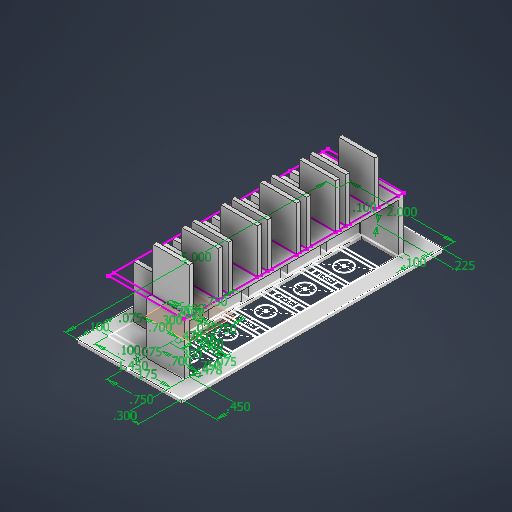
# Autodesk Inventor part: SolenoidHolders
Saved by Autodesk Inventor 2026.2 (Build 302298010, 298A)
## iProperties
Created: 2026-03-29
Part Number: SolenoidHolders
Material: Generic
Document SubType Name: Modeling
Designer: david
Density: 1 g/cm^3
Appearance: Default
Author: david
Autodesk Inventor part; units mm, degrees
ref_plane "YZ Plane" through (0, 0, 0) normal (1, 0, 0) x (0, 1, 0)
ref_plane "XZ Plane" through (0, 0, 0) normal (0, 1, 0) x (-1, 0, 0)
ref_plane "XY Plane" through (0, 0, 0) normal (0, 0, 1) x (1, 0, 0)
sketch "Sketch2" plane through (0, 0, 0) normal (0, 1, 0) x (-1, 0, 0)
  line L0 (0, 0) -> (17.78, 0)
  line L1 (17.78, 0) -> (17.78, -1.905)
  line L2 (17.78, -1.905) -> (0, -1.905)
  line L3 (0, -1.905) -> (0, 0)
  line L4 (17.78, -1.905) -> (0, -1.905)
  line L5 (0, -1.905) -> (0, -14.0462)
  line L6 (0, -14.0462) -> (17.78, -14.0462)
  line L7 (17.78, -14.0462) -> (17.78, -1.905)
  line L8 (17.78, -14.0462) -> (0, -14.0462)
  line L9 (0, -14.0462) -> (0, -15.9512)
  line L10 (0, -15.9512) -> (17.78, -15.9512)
  line L11 (17.78, -15.9512) -> (17.78, -14.0462)
  circle A0 centre (8.89, -7.9756) radius 3.81
  line L12 (17.78, -1.905) -> (0, -14.0462) construction
  line L13 (0, -19.05) -> (17.78, -19.05)
  line L14 (17.78, -19.05) -> (17.78, -20.955)
  line L15 (17.78, -20.955) -> (0, -20.955)
  line L16 (0, -20.955) -> (0, -19.05)
  line L17 (17.78, -20.955) -> (0, -20.955)
  line L18 (0, -20.955) -> (0, -33.0962)
  line L19 (0, -33.0962) -> (17.78, -33.0962)
  line L20 (17.78, -33.0962) -> (17.78, -20.955)
  line L21 (17.78, -33.0962) -> (0, -33.0962)
  line L22 (0, -33.0962) -> (0, -35.0012)
  line L23 (0, -35.0012) -> (17.78, -35.0012)
  line L24 (17.78, -35.0012) -> (17.78, -33.0962)
  circle A1 centre (8.89, -27.0256) radius 3.81
  line L25 (17.78, -20.955) -> (0, -33.0962) construction
  line L26 (0, -38.1) -> (17.78, -38.1)
  line L27 (17.78, -38.1) -> (17.78, -40.005)
  line L28 (17.78, -40.005) -> (0, -40.005)
  line L29 (0, -40.005) -> (0, -38.1)
  line L30 (17.78, -40.005) -> (0, -40.005)
  line L31 (0, -40.005) -> (0, -52.1462)
  line L32 (0, -52.1462) -> (17.78, -52.1462)
  line L33 (17.78, -52.1462) -> (17.78, -40.005)
  line L34 (17.78, -52.1462) -> (0, -52.1462)
  line L35 (0, -52.1462) -> (0, -54.0512)
  line L36 (0, -54.0512) -> (17.78, -54.0512)
  line L37 (17.78, -54.0512) -> (17.78, -52.1462)
  circle A2 centre (8.89, -46.0756) radius 3.81
  line L38 (17.78, -40.005) -> (0, -52.1462) construction
  line L39 (0, -57.15) -> (17.78, -57.15)
  line L40 (17.78, -57.15) -> (17.78, -59.055)
  line L41 (17.78, -59.055) -> (0, -59.055)
  line L42 (0, -59.055) -> (0, -57.15)
  line L43 (17.78, -59.055) -> (0, -59.055)
  line L44 (0, -59.055) -> (0, -71.1962)
  line L45 (0, -71.1962) -> (17.78, -71.1962)
  line L46 (17.78, -71.1962) -> (17.78, -59.055)
  line L47 (17.78, -71.1962) -> (0, -71.1962)
  line L48 (0, -71.1962) -> (0, -73.1012)
  line L49 (0, -73.1012) -> (17.78, -73.1012)
  line L50 (17.78, -73.1012) -> (17.78, -71.1962)
  circle A3 centre (8.89, -65.1256) radius 3.81
  line L51 (17.78, -59.055) -> (0, -71.1962) construction
  line L52 (0, -76.2) -> (17.78, -76.2)
  line L53 (17.78, -76.2) -> (17.78, -78.105)
  line L54 (17.78, -78.105) -> (0, -78.105)
  line L55 (0, -78.105) -> (0, -76.2)
  line L56 (17.78, -78.105) -> (0, -78.105)
  line L57 (0, -78.105) -> (0, -90.2462)
  line L58 (0, -90.2462) -> (17.78, -90.2462)
  line L59 (17.78, -90.2462) -> (17.78, -78.105)
  line L60 (17.78, -90.2462) -> (0, -90.2462)
  line L61 (0, -90.2462) -> (0, -92.1512)
  line L62 (0, -92.1512) -> (17.78, -92.1512)
  line L63 (17.78, -92.1512) -> (17.78, -90.2462)
  circle A4 centre (8.89, -84.1756) radius 3.81
  line L64 (17.78, -78.105) -> (0, -90.2462) construction
  line L65 (-7.62, 11.43) -> (43.18, 11.43)
  line L66 (43.18, 11.43) -> (43.18, -115.57)
  line L67 (43.18, -115.57) -> (-7.62, -115.57)
  line L68 (-7.62, -115.57) -> (-7.62, 11.43)
  line L69 (19.05, -9.525) -> (36.83, -9.525)
  line L70 (36.83, -9.525) -> (36.83, -11.43)
  line L71 (36.83, -11.43) -> (19.05, -11.43)
  line L72 (19.05, -11.43) -> (19.05, -9.525)
  line L73 (36.83, -11.43) -> (19.05, -11.43)
  line L74 (19.05, -11.43) -> (19.05, -23.5712)
  line L75 (19.05, -23.5712) -> (36.83, -23.5712)
  line L76 (36.83, -23.5712) -> (36.83, -11.43)
  line L77 (36.83, -23.5712) -> (19.05, -23.5712)
  line L78 (19.05, -23.5712) -> (19.05, -25.4762)
  line L79 (19.05, -25.4762) -> (36.83, -25.4762)
  line L80 (36.83, -25.4762) -> (36.83, -23.5712)
  circle A5 centre (27.94, -17.5006) radius 3.81
  line L81 (36.83, -11.43) -> (19.05, -23.5712) construction
  line L82 (19.05, -28.575) -> (36.83, -28.575)
  line L83 (36.83, -28.575) -> (36.83, -30.48)
  line L84 (36.83, -30.48) -> (19.05, -30.48)
  line L85 (19.05, -30.48) -> (19.05, -28.575)
  line L86 (36.83, -30.48) -> (19.05, -30.48)
  line L87 (19.05, -30.48) -> (19.05, -42.6212)
  line L88 (19.05, -42.6212) -> (36.83, -42.6212)
  line L89 (36.83, -42.6212) -> (36.83, -30.48)
  line L90 (36.83, -42.6212) -> (19.05, -42.6212)
  line L91 (19.05, -42.6212) -> (19.05, -44.5262)
  line L92 (19.05, -44.5262) -> (36.83, -44.5262)
  line L93 (36.83, -44.5262) -> (36.83, -42.6212)
  circle A6 centre (27.94, -36.5506) radius 3.81
  line L94 (36.83, -30.48) -> (19.05, -42.6212) construction
  line L95 (19.05, -47.625) -> (36.83, -47.625)
  line L96 (36.83, -47.625) -> (36.83, -49.53)
  line L97 (36.83, -49.53) -> (19.05, -49.53)
  line L98 (19.05, -49.53) -> (19.05, -47.625)
  line L99 (36.83, -49.53) -> (19.05, -49.53)
  line L100 (19.05, -49.53) -> (19.05, -61.6712)
  line L101 (19.05, -61.6712) -> (36.83, -61.6712)
  line L102 (36.83, -61.6712) -> (36.83, -49.53)
  line L103 (36.83, -61.6712) -> (19.05, -61.6712)
  line L104 (19.05, -61.6712) -> (19.05, -63.5762)
  line L105 (19.05, -63.5762) -> (36.83, -63.5762)
  line L106 (36.83, -63.5762) -> (36.83, -61.6712)
  circle A7 centre (27.94, -55.6006) radius 3.81
  line L107 (36.83, -49.53) -> (19.05, -61.6712) construction
  line L108 (19.05, -66.675) -> (36.83, -66.675)
  line L109 (36.83, -66.675) -> (36.83, -68.58)
  line L110 (36.83, -68.58) -> (19.05, -68.58)
  line L111 (19.05, -68.58) -> (19.05, -66.675)
  line L112 (36.83, -68.58) -> (19.05, -68.58)
  line L113 (19.05, -68.58) -> (19.05, -80.7212)
  line L114 (19.05, -80.7212) -> (36.83, -80.7212)
  line L115 (36.83, -80.7212) -> (36.83, -68.58)
  line L116 (36.83, -80.7212) -> (19.05, -80.7212)
  line L117 (19.05, -80.7212) -> (19.05, -82.6262)
  line L118 (19.05, -82.6262) -> (36.83, -82.6262)
  line L119 (36.83, -82.6262) -> (36.83, -80.7212)
  circle A8 centre (27.94, -74.6506) radius 3.81
  line L120 (36.83, -68.58) -> (19.05, -80.7212) construction
  line L121 (19.05, -85.725) -> (36.83, -85.725)
  line L122 (36.83, -85.725) -> (36.83, -87.63)
  line L123 (36.83, -87.63) -> (19.05, -87.63)
  line L124 (19.05, -87.63) -> (19.05, -85.725)
  line L125 (36.83, -87.63) -> (19.05, -87.63)
  line L126 (19.05, -87.63) -> (19.05, -99.7712)
  line L127 (19.05, -99.7712) -> (36.83, -99.7712)
  line L128 (36.83, -99.7712) -> (36.83, -87.63)
  line L129 (36.83, -99.7712) -> (19.05, -99.7712)
  line L130 (19.05, -99.7712) -> (19.05, -101.6762)
  line L131 (19.05, -101.6762) -> (36.83, -101.6762)
  line L132 (36.83, -101.6762) -> (36.83, -99.7712)
  circle A9 centre (27.94, -93.7006) radius 3.81
  line L133 (36.83, -87.63) -> (19.05, -99.7712)
  line L134 (8.89, -15.9512) -> (8.89, -19.05) construction
  line L135 (0, 0) -> (36.83, 0)
  line L136 (36.83, 0) -> (36.83, 2.54)
  line L137 (36.83, 2.54) -> (0, 2.54)
  line L138 (0, 2.54) -> (0, 0)
  line L139 (36.83, -101.6762) -> (0, -101.6762)
  line L140 (0, -101.6762) -> (0, -104.2162)
  line L141 (0, -104.2162) -> (36.83, -104.2162)
  line L142 (36.83, -104.2162) -> (36.83, -101.6762)
  circle A10 centre (18.415, 6.985) radius 1.27
  line L143 (19.05, -9.525) -> (17.78, -9.525) construction
  line L144 (19.05, -10.4775) -> (17.78, -10.4775) construction
  circle A11 centre (18.415, -109.855) radius 1.27
  line L145 (22.86, -25.4762) -> (22.86, -28.575)
  line L146 (22.86, -28.575) -> (33.02, -28.575)
  line L147 (33.02, -28.575) -> (33.02, -25.4762)
  line L148 (33.02, -25.4762) -> (22.86, -25.4762)
  line L149 (22.86, -25.4762) -> (33.02, -28.575) construction
  line L150 (22.86, -28.575) -> (33.02, -25.4762) construction
  line L151 (22.86, -47.625) -> (33.02, -47.625)
  line L152 (33.02, -44.5262) -> (22.86, -44.5262)
  line L153 (22.86, -44.5262) -> (22.86, -47.625)
  line L154 (33.02, -47.625) -> (33.02, -44.5262)
  line L155 (22.86, -44.5262) -> (33.02, -47.625) construction
  line L156 (22.86, -47.625) -> (33.02, -44.5262) construction
  line L157 (22.86, -66.675) -> (33.02, -66.675)
  line L158 (33.02, -63.5762) -> (22.86, -63.5762)
  line L159 (22.86, -63.5762) -> (22.86, -66.675)
  line L160 (33.02, -66.675) -> (33.02, -63.5762)
  line L161 (22.86, -63.5762) -> (33.02, -66.675) construction
  line L162 (22.86, -66.675) -> (33.02, -63.5762) construction
  line L163 (22.86, -85.725) -> (33.02, -85.725)
  line L164 (33.02, -82.6262) -> (22.86, -82.6262)
  line L165 (22.86, -82.6262) -> (22.86, -85.725)
  line L166 (33.02, -85.725) -> (33.02, -82.6262)
  line L167 (22.86, -82.6262) -> (33.02, -85.725) construction
  line L168 (22.86, -85.725) -> (33.02, -82.6262) construction
  line L169 (3.81, -15.9512) -> (3.81, -19.05)
  line L170 (3.81, -19.05) -> (13.97, -19.05)
  line L171 (13.97, -19.05) -> (13.97, -15.9512)
  line L172 (13.97, -15.9512) -> (3.81, -15.9512)
  line L173 (3.81, -15.9512) -> (13.97, -19.05) construction
  line L174 (3.81, -19.05) -> (13.97, -15.9512) construction
  line L175 (3.81, -38.1) -> (13.97, -38.1)
  line L176 (13.97, -35.0012) -> (3.81, -35.0012)
  line L177 (3.81, -35.0012) -> (13.97, -38.1) construction
  line L178 (3.81, -38.1) -> (13.97, -35.0012) construction
  line L179 (3.81, -35.0012) -> (3.81, -38.1)
  line L180 (13.97, -38.1) -> (13.97, -35.0012)
  line L181 (8.89, -35.0012) -> (8.89, -38.1) construction
  line L182 (3.81, -57.15) -> (13.97, -57.15)
  line L183 (13.97, -54.0512) -> (3.81, -54.0512)
  line L184 (3.81, -54.0512) -> (13.97, -57.15) construction
  line L185 (3.81, -57.15) -> (13.97, -54.0512) construction
  line L186 (3.81, -54.0512) -> (3.81, -57.15)
  line L187 (13.97, -57.15) -> (13.97, -54.0512)
  line L188 (8.89, -54.0512) -> (8.89, -57.15) construction
  line L189 (3.81, -76.2) -> (13.97, -76.2)
  line L190 (13.97, -73.1012) -> (3.81, -73.1012)
  line L191 (3.81, -73.1012) -> (13.97, -76.2) construction
  line L192 (3.81, -76.2) -> (13.97, -73.1012) construction
  line L193 (3.81, -73.1012) -> (3.81, -76.2)
  line L194 (13.97, -76.2) -> (13.97, -73.1012)
  line L195 (8.89, -73.1012) -> (8.89, -76.2) construction
  line L196 (0, 0) -> (17.78, 0)
  line L197 (17.78, 0) -> (17.78, -101.6762)
  line L198 (17.78, -101.6762) -> (0, -101.6762)
  line L199 (0, -101.6762) -> (0, 0)
  line L200 (36.83, 0) -> (0, 0)
  line L201 (0, 0) -> (0, -101.6762)
  line L202 (0, -101.6762) -> (36.83, -101.6762)
  line L203 (36.83, -101.6762) -> (36.83, 0)
  line L204 (18.415, 2.54) -> (18.415, 0)
  line L205 (18.415, -101.6762) -> (18.415, -104.2162)
  point P0 (8.89, -17.5006)
  point P1 (18.415, -10.4775)
  point P2 (17.78, 11.43)
  point P3 (31.0864, -91.5521)
  point P4 (24.7936, -95.8491)
  point P5 (27.94, -27.0256)
  point P6 (27.94, -27.0256)
  point P7 (27.94, -46.0756)
  point P8 (27.94, -46.0756)
  point P9 (27.94, -65.1256)
  point P10 (27.94, -65.1256)
  point P11 (27.94, -84.1756)
  point P12 (27.94, -84.1756)
  point P13 (8.89, -36.5506)
  point P14 (8.89, -55.6006)
  point P15 (8.89, -74.6506)
  dimension "d68" = 17.78
  dimension "d69" = 1.905
  dimension "d70" = 17.78
  dimension "d71" = 12.1412
  dimension "d72" = 17.78
  dimension "d73" = 1.905
  dimension "d74" = 7.62
  dimension "d77" = 19.05
  dimension "d82" = 50.8
  dimension "d83" = 127
  dimension "d84" = 11.43
  dimension "d85" = 7.62
  dimension "d90" = 17.78
  dimension "d91" = 1.905
  dimension "d92" = 17.78
  dimension "d93" = 12.1412
  dimension "d94" = 17.78
  dimension "d95" = 1.905
  dimension "d96" = 7.62
  dimension "d97" = 19.05
  dimension "d99" = 19.05
  dimension "d100" = 36.83
  dimension "d101" = 2.54
  dimension "d102" = 2.54
  dimension "d103" = 2.54
  dimension "d104" = 4.445
  dimension "d105" = 2.54
  dimension "d106" = 5.715
  dimension "d113" = 10.16
  dimension "d114" = 3.0988
  dimension "d117" = 19.05
  dimension "d122" = 10.16
  dimension "d125" = 19.05
  constraints: 412 end point, 29 midpoint, 26 parallel, 17 perpendicular, 12 centre point, 11 horizontal, 10 coincident, 6 collinear, 4 vertical, 3 point on line, 3 vertical alignment, 1 horizontal alignment, 284 other
  measures "d68" distance of L1.end L2.end
  measures "d69" distance of L0.end L1.end
  measures "d70" distance of L6.end L5.end
  measures "d71" distance of L5.end L4.end
  measures "d72" distance of L10.end L9.end
  measures "d73" distance of L9.end L8.end
  measures "d74" diameter of A0
  measures "d77" distance of L0.start L13.start
  measures "d82" distance of L66.end L67.end
  measures "d83" distance of L65.end L66.end
  measures "d84" distance between parallel lines of L0 L65
  measures "d85" distance from line of L0.start L68
  measures "d90" distance of L71.start L71.end
  measures "d91" distance of L69.end L71.start
  measures "d92" distance of L75.end L74.end
  measures "d93" distance of L74.end L73.end
  measures "d94" distance of L79.end L78.end
  measures "d95" distance of L78.end L77.end
  measures "d96" diameter of A5
  measures "d97" distance of L69.start L82.start
  measures "d99" distance between parallel lines of L18 L74
  measures "d100" distance of L137.end L136.end
  measures "d101" distance of L136.end L135.end
  measures "d102" distance of L140.end L139.end
  measures "d103" diameter of A10
  measures "d104" vertical distance of point (17.78, 11.43) A10.centre
  measures "d105" diameter of A11
  measures "d106" distance from line of L67 A11.centre
  measures "d113" distance of L146.end L145.end
  measures "d114" distance between parallel lines of L146 L148
  measures "d117" distance of L145.end L151.start
  measures "d122" distance of L170.end L169.end
  measures "d125" distance of L170.end L175.end
extrude "Extrusion1" add sketch "Sketch2" against normal blind 1.905 contours L138 L137 L204 L135 L0 | L135 L203 L69 L72 L74 L78 L79 L145 L82 L85 L87 L91 L92 L153 L95 L98 L100 L104 L105 L159 L108 L111 L113 L117 L118 L165 L121 L124 L126 L130 L139 L197 L63 L59 L53 L50 L46 L40 L37 L33 L27 L24 L20 L14 L11 L7 L1 | L204 L137 L136 L135 | L70 L71 L72 L69 | L76 L75 L74 L71 | L80 L79 L78 L75 | L203 L82 L147 L79 | L147 L82 L145 L79 | L83 L84 L85 L82 | L89 L88 L87 L84 | L93 L92 L91 L88 | L203 L95 L154 L92 | L154 L95 L153 L92 | L96 L97 L98 L95 | L102 L101 L100 L97 | L106 L105 L104 L101 | L203 L108 L160 L105 | L160 L108 L159 L105 | L109 L110 L111 L108 | L115 L114 L113 L110 | L119 L118 L117 L114 | L203 L121 L166 L118 | L166 L121 L165 L118 | L122 L123 L124 L121 | L139 L205 L141 L140 | L133 A9 L126 L123 | L128 L127 L133 A9 | L139 L131 L142 L141 L205 | L132 L131 L130 L127 | L133 A9 | A9 L133 | L65 L66 L67 L68 | A5 | A6 | A7 | A8
extrude "Extrusion2" add sketch "Sketch2" along normal blind 6.985 contours L76 L75 L74 L71 | L89 L88 L87 L84 | L102 L101 L100 L97 | L115 L114 L113 L110 | L133 A9 L126 L123 | L128 L127 L133 A9 | L133 A9 | A9 L133 | A5 | A6 | A7 | A8
extrude "Extrusion3" add sketch "Sketch2" along normal blind 25.4 contours L70 L71 L72 L69 | L80 L79 L78 L75 | L83 L84 L85 L82 | L93 L92 L91 L88 | L96 L97 L98 L95 | L106 L105 L104 L101 | L109 L110 L111 L108 | L119 L118 L117 L114 | L122 L123 L124 L121 | L132 L131 L130 L127
extrude "Extrusion4" add sketch "Sketch2" along normal blind 20.32 contours L147 L82 L145 L79 | L154 L95 L153 L92 | L160 L108 L159 L105 | L166 L121 L165 L118
ref_plane "Work Plane1" through (0, 25.4, 0) normal (0, 1, 0) x (1, 0, 0)
sketch "Sketch3" plane through (0, 25.4, 0) normal (0, 1, 0) x (1, 0, 0)
  line L0 (-36.83, 101.6762) -> (-36.83, 0) projected
  line L1 (0, 0) -> (-36.83, 0) projected
  line L2 (0, 101.6762) -> (0, 0) projected
  line L3 (-19.05, 101.6762) -> (0, 101.6762) projected
  line L4 (-19.05, 101.6762) -> (-36.83, 101.6762) projected
  line L5 (0, 0) -> (-17.78, 0) projected
  line L6 (-17.78, 0) -> (-17.78, 101.6762) projected
  line L7 (-17.78, 1.905) -> (0, 1.905) projected
  line L8 (-17.78, 14.0462) -> (0, 14.0462) projected
  line L9 (0, 15.9512) -> (-17.78, 15.9512) projected
  line L10 (0, 19.05) -> (-17.78, 19.05) projected
  line L11 (-17.78, 20.955) -> (0, 20.955) projected
  line L12 (-17.78, 33.0962) -> (0, 33.0962) projected
  line L13 (0, 35.0012) -> (-17.78, 35.0012) projected
  line L14 (-3.81, 35.0012) -> (-3.81, 38.1) projected
  line L15 (-13.97, 38.1) -> (-13.97, 35.0012) projected
  line L16 (0, 38.1) -> (-17.78, 38.1) projected
  line L17 (-17.78, 40.005) -> (0, 40.005) projected
  line L18 (-17.78, 52.1462) -> (0, 52.1462) projected
  line L19 (0, 54.0512) -> (-17.78, 54.0512) projected
  line L20 (0, 57.15) -> (-17.78, 57.15) projected
  line L21 (-17.78, 59.055) -> (0, 59.055) projected
  line L22 (0, 71.1962) -> (-17.78, 71.1962) projected
  line L23 (0, 73.1012) -> (-17.78, 73.1012) projected
  line L24 (0, 76.2) -> (-17.78, 76.2) projected
  line L25 (-17.78, 78.105) -> (0, 78.105) projected
  line L26 (0, 90.2462) -> (-17.78, 90.2462) projected
  line L27 (0, 92.1512) -> (-17.78, 92.1512) projected
  line L28 (-13.97, 76.2) -> (-13.97, 73.1012) projected
  line L29 (-3.81, 73.1012) -> (-3.81, 76.2) projected
  line L30 (-13.97, 57.15) -> (-13.97, 54.0512) projected
  line L31 (-3.81, 54.0512) -> (-3.81, 57.15) projected
  line L32 (0, -2.54) -> (-36.83, -2.54) projected
  line L33 (-36.83, 104.2162) -> (0, 104.2162) projected
  line L34 (-36.83, 85.725) -> (-36.83, 104.2162) projected
  line L35 (0, 101.6762) -> (0, 104.2162) projected
  line L36 (0, -2.54) -> (0, 0) projected
  line L37 (-13.97, 19.05) -> (-13.97, 15.9512) projected
  line L38 (-3.81, 15.9512) -> (-3.81, 19.05) projected
  line L39 (-36.83, -2.54) -> (-36.83, 0) projected
  constraints: 2 other
extrude "Extrusion6" add sketch "Sketch3" against normal blind 1.905 contours L3 L2 L27 L6 | L6 L7 L2 L1 | L27 L2 L26 L6 | L6 L8 L2 L7 | L26 L2 L25 L6 | L6 L9 L2 L8 | L25 L2 L24 L6 | L6 L10 L37 L9 | L24 L28 L23 L6 | L9 L38 L10 L2 | L6 L11 L2 L10 | L37 L10 L38 L9 | L2 L23 L29 L24 | L23 L2 L22 L6 | L24 L29 L23 L28 | L6 L12 L2 L11 | L22 L2 L21 L6 | L6 L13 L2 L12 | L21 L2 L20 L6 | L6 L16 L15 L13 | L20 L30 L19 L6 | L13 L14 L16 L2 | L6 L17 L2 L16 | L15 L16 L14 L13 | L2 L19 L31 L20 | L19 L2 L18 L6 | L20 L31 L19 L30 | L6 L18 L2 L17
extrude "Extrusion7" add sketch "Sketch2" along normal blind 25.4 contours L138 L137 L204 L135 L0 | L139 L205 L141 L140
sketch "Sketch4" plane through (0, 25.4, 0) normal (0, 1, 0) x (1, 0, 0)
  point P0 (0, 0)
extrude "Extrusion8" add sketch "Sketch3" along normal blind 21.59 contours L6 L7 L2 L1 | L27 L2 L26 L6 | L6 L9 L2 L8 | L25 L2 L24 L6 | L6 L11 L2 L10 | L23 L2 L22 L6 | L6 L13 L2 L12 | L21 L2 L20 L6 | L6 L17 L2 L16 | L19 L2 L18 L6
extrude "Extrusion9" add sketch "Sketch3" along normal blind 16.51 contours L37 L10 L38 L9 | L24 L29 L23 L28 | L15 L16 L14 L13 | L20 L31 L19 L30
body "Solid1"
